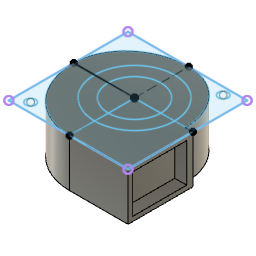
air_mask_vortex v19 (Autodesk Fusion 360 archive; units mm, degrees)
design "fan_1"
Autodesk Fusion 360 part; units mm, degrees
sketch "草图1" plane through (0, 0, 0) normal (0, 0, 1) x (1, 0, 0)
  circle A0 centre (-13.6473, 1.2662) radius 16.75
  circle A1 centre (-13.6473, 1.2662) radius 11
  circle A2 centre (3.8527, 20.9662) radius 2
  circle A3 centre (-33.9473, -22.0338) radius 2
  line L0 (10.8527, -25.9797) -> (-13.6473, -25.9797)
  line L1 (-13.6473, -25.9797) -> (-13.6473, 1.2662)
  line L2 (-13.6473, 1.2662) -> (10.8527, 1.2662)
  line L3 (10.8527, 1.2662) -> (10.8527, -25.9797)
  line L4 (10.8527, -25.9797) -> (-39.1473, -25.9797)
  line L5 (-39.1473, -25.9797) -> (-39.1473, 24.0203)
  line L6 (-39.1473, 24.0203) -> (10.8527, 24.0203)
  line L7 (10.8527, 24.0203) -> (10.8527, -25.9797)
  dimension "d1" = 33.5
  dimension "d2" = 22
  dimension "d3" = 19.7
  dimension "d4" = 17.5
  dimension "d5" = 4
  dimension "d6" = 20.3
  dimension "d7" = 23.3
  dimension "d8" = 4
  dimension "d9" = 24.5
  dimension "d11" = 50
  dimension "d12" = 50
  constraint concentric A0 A1
  constraint horizontal L0
  constraint vertical L1
  constraint horizontal L2
  constraint vertical L3
  constraint coincident A0.centre A1.centre
  constraint horizontal L4
  constraint vertical L5
  constraint horizontal L6
  constraint vertical L7
  measures "d1" diameter of A0
  measures "d2" diameter of A1
  measures "d3" vertical distance of A0.centre A2.centre
  measures "d4" horizontal distance of A0.centre A2.centre
  measures "d5" diameter of A2
  measures "d6" horizontal distance of A0.centre A3.centre
  measures "d7" vertical distance of A0.centre A3.centre
  measures "d8" diameter of A3
  measures "d9" distance of L0.start L0.end
  measures "d11" distance of L0.start L4.end
  measures "d12" distance of L0.start L6.end
sketch "草图2" plane through (0, 0, 0) normal (0, 0, 1) x (1, 0, 0)
  line L0 (10.8527, 24.0203) -> (10.8527, -25.9797)
  line L1 (-39.1473, 24.0203) -> (10.8527, 24.0203)
  line L2 (-39.1473, -25.9797) -> (-39.1473, 24.0203)
  line L3 (10.8527, -25.9797) -> (-39.1473, -25.9797)
  line L4 (-13.6473, 1.2662) -> (-13.6473, 24.0203) construction
  line L5 (-13.6473, 1.2662) -> (10.8527, 1.2662) construction
  line L6 (-13.6473, 1.2662) -> (-39.1473, 1.2662) construction
  line L7 (-39.1473, 1.2662) -> (-13.6473, 1.2662)
  line L8 (-13.6473, -25.9797) -> (-13.6473, 1.2662) construction
  ellipse E0 centre (-13.6473, 1.2662) end of major axis (-13.6473, 24.0203) minor radius 21.4054 (7.7581, 1.2662) -> (-13.6473, 24.0203) ccw
  ellipse E1 centre (-13.6473, 1.2662) end of major axis (-13.6473, 24.0203) minor radius 25.5 (-13.6473, 24.0203) -> (-39.1473, 1.2662) ccw
  ellipse E2 centre (-13.6473, 1.2662) end of major axis (-39.1473, 1.2662) minor radius 27.2458 (-39.1473, 1.2662) -> (-13.6473, -25.9797) ccw
  line L9 (10.8527, 1.2662) -> (7.7581, 1.2662)
  point P0 (-13.6473, 1.2662)
  constraint coincident P0 L4.start
  constraint coincident L1 L4.end
  constraint perpendicular L1 L4
  constraint coincident L0 L5.end
  constraint perpendicular L0 L5
  constraint coincident L2 L6.end
  constraint perpendicular L2 L6
  constraint coincident L3 L8.start
  constraint vertical L8
  constraint coincident L5 L9.end
  constraint concentric E0 E2
extrude "拉伸1" add sketch "草图2" against normal blind 20 contours L0 L3 E0 E1 E2 L9
sketch "草图3" plane through (10.8527, 0, 0) normal (1, 0, 0) x (0, 1, 0)
  line L0 (1.2662, 0) -> (-25.9797, 0)
  line L1 (-25.9797, 0) -> (-25.9797, -20)
  line L2 (-25.9797, -20) -> (1.2662, -20)
  line L3 (1.2662, -20) -> (1.2662, 0)
  line L4 (-24.0386, -1.9) -> (-1.3386, -1.9)
  line L5 (-1.3386, -1.9) -> (-1.3386, -18.1)
  line L6 (-1.3386, -18.1) -> (-24.0386, -18.1)
  line L7 (-24.0386, -18.1) -> (-24.0386, -1.9)
  point P0 (-1.3386, -10)
  point P1 (1.2662, -10)
  point P2 (-12.3567, 0)
  point P3 (-12.6886, -1.9)
  dimension "d15" = 22.7
  dimension "d16" = 16.2
  constraint horizontal L4
  constraint vertical L5
  constraint horizontal L6
  constraint vertical L7
  constraint midpoint L5 P0
  constraint midpoint L3 P1
  constraint midpoint L0 P2
  constraint midpoint L4 P3
  constraint horizontal P0 P1
  measures "d15" distance of L4.start L4.end
  measures "d16" distance of L4.end L5.end
extrude "拉伸2" cut sketch "草图3" against normal blind 5 contours L4 L5 L6 L7
